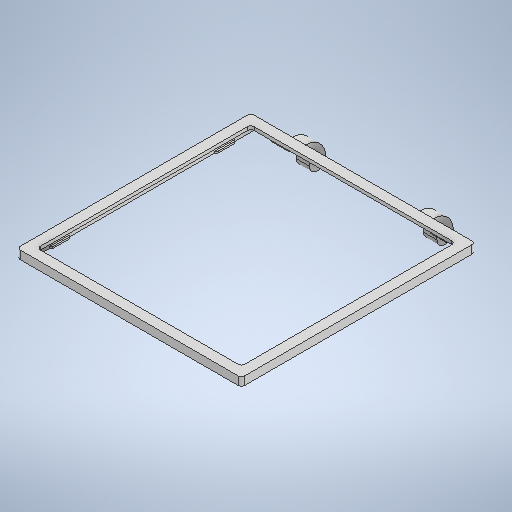
# Autodesk Inventor part: Pieza4
Saved by Autodesk Inventor 2025.1 (Build 291241000, 241)
## iProperties
Created: 2024-08-13
Part Number: Pieza4
Material: Genérico
Document SubType Name: Modeling
Designer: andre
Density: 1 g/cm^3
Appearance: Valor por defecto
Author: andre
Autodesk Inventor part; units mm, degrees
ref_plane "YZ Plane" through (0, 0, 0) normal (1, 0, 0) x (0, 1, 0)
ref_plane "XZ Plane" through (0, 0, 0) normal (0, 1, 0) x (-1, 0, 0)
ref_plane "XY Plane" through (0, 0, 0) normal (0, 0, 1) x (1, 0, 0)
sketch "Boceto1" plane through (0, 0, 0) normal (0, 1, 0) x (-1, 0, 0)
  line L0 (2, 0) -> (132.4, 0)
  line L1 (134.4, -2) -> (134.4, -138)
  line L2 (132.4, -140) -> (2, -140)
  line L3 (0, -138) -> (0, -2)
  arc A0 (134.4, -2) -> (132.4, 0) centre (132.4, -2) ccw
  arc A1 (132.4, -140) -> (134.4, -138) centre (132.4, -138) ccw
  arc A2 (0, -138) -> (2, -140) centre (2, -138) ccw
  arc A3 (2, 0) -> (0, -2) centre (2, -2) ccw
  line L4 (126.4, -6) -> (8, -6)
  line L5 (6, -8) -> (6, -132)
  line L6 (8, -134) -> (126.4, -134)
  line L7 (128.4, -132) -> (128.4, -8)
  arc A4 (8, -6) -> (6, -8) centre (8, -8) ccw
  arc A5 (6, -132) -> (8, -134) centre (8, -132) ccw
  arc A6 (126.4, -134) -> (128.4, -132) centre (126.4, -132) ccw
  arc A7 (128.4, -8) -> (126.4, -6) centre (126.4, -8) ccw
  line L8 (67.2, -140) -> (67.2, 0) construction
  line L9 (134.4, -140) -> (109.4, -140) construction
  line L10 (109.4, -140) -> (101.4, -140) construction
  line L11 (101.4, -140) -> (101.4, -152)
  line L12 (101.4, -152) -> (109.4, -152)
  line L13 (109.4, -152) -> (109.4, -140)
  line L14 (0, -140) -> (25, -140) construction
  line L15 (25, -140) -> (33, -140) construction
  line L16 (33, -140) -> (33, -152)
  line L17 (33, -152) -> (25, -152)
  line L18 (25, -152) -> (25, -140)
  point P0 (0, 0)
  point P1 (134.4, 0)
  point P2 (25, -140)
  point P3 (101.4, -140)
  dimension "d0" = 134.4
  dimension "d1" = 140
  dimension "d2" = 2
  dimension "d3" = 6
  dimension "d4" = 2
  dimension "d7" = 25
  dimension "d8" = 8
  dimension "d9" = 12
  constraints: 38 end point, 16 point on circle, 16 tangent, 9 point on line, 8 centre point, 6 equal radius, 6 parallel, 4 symmetric about line, 3 perpendicular, 2 horizontal, 2 midpoint, 3 other
  measures "d0" distance of L9.start L14.start
  measures "d1" distance of point (134.4, 0) L9.start
  measures "d2" radius of A0
  measures "d3" distance between parallel lines of L0 L4
  measures "d4" radius of A4
  measures "d7" distance of L9.start L9.end
  measures "d8" distance of L12.end L11.end
  measures "d9" distance of L11.end L10.end
extrude "Extrusión1" add sketch "Boceto1" along normal blind 5
sketch "Boceto2" plane through (0, 0, 0) normal (0, -1, 0) x (1, 0, 0)
  line L0 (-25, -140) -> (-25, -152) projected
  line L1 (-33, -140) -> (-101.4, -140) projected
  line L2 (-25, -152) -> (-33, -152)
  line L3 (-33, -152) -> (-33, -140)
  line L4 (-33, -140) -> (-25, -140)
  line L5 (-25, -140) -> (-25, -152)
  line L6 (-101.4, -152) -> (-109.4, -152) projected
  line L7 (-109.4, -152) -> (-101.4, -152)
  line L8 (-101.4, -152) -> (-101.4, -140)
  line L9 (-101.4, -140) -> (-109.4, -140)
  line L10 (-109.4, -140) -> (-109.4, -152)
  line L11 (-109.4, -140) -> (-101.4, -140)
  line L12 (-101.4, -140) -> (-101.4, -136)
  line L13 (-101.4, -136) -> (-109.4, -136)
  line L14 (-109.4, -136) -> (-109.4, -140)
  line L15 (-33, -140) -> (-25, -140)
  line L16 (-25, -140) -> (-25, -136)
  line L17 (-25, -136) -> (-33, -136)
  line L18 (-33, -136) -> (-33, -140)
  point P0 (0, 0)
  dimension "d18" = 4
  dimension "d19" = 8
  dimension "d20" = 4
  constraints: 32 end point, 8 parallel, 4 horizontal, 4 perpendicular
  measures "d18" distance of L12.end L11.end
  measures "d19" distance of L17.end L16.end
  measures "d20" distance of L16.end L15.end
extrude "Extrusión2" add sketch "Boceto2" along normal blind 18
sketch "Boceto3" plane through (-109.4, 5, -152) normal (-1, 0, 0) x (0, 0, 1)
  line L0 (14, -5) -> (12, -5) construction
  line L1 (0, -23) -> (0, 0) projected
  line L2 (12, -5) -> (0, -5) construction
  line L3 (0, -5) -> (0, -12) construction
  line L4 (12, -12) -> (12, -5) construction
  circle A0 centre (5, -12) radius 2.125
  circle A1 centre (5, -12) radius 4.875 construction
  arc A2 (0.125, -12) -> (9.875, -12) centre (5, -12) ccw
  line L5 (0.125, -12) -> (0.125, 0) construction
  line L6 (12, 0) -> (0, 0) construction
  line L7 (12, -5) -> (12, 0) construction
  line L8 (9.8743, -12.0803) -> (9.8743, -5) construction
  line L9 (12, -5) -> (5, -5) construction
  line L10 (5, -5) -> (5, -12) construction
  line L11 (5, -12) -> (12, -12) construction
  line L12 (12, -12) -> (12, -5) construction
  line L13 (14, -5) -> (14, -23) construction
  line L14 (16, -23) -> (0, -23) projected
  line L15 (12, -5) -> (14, -5) construction
  line L16 (14, -5) -> (14, -7) construction
  line L17 (14, -7) -> (12, -7) construction
  line L18 (12, -7) -> (12, -5) construction
  arc A3 (14, -5) -> (12, -7) centre (14, -7) ccw construction
  line L19 (14, 0) -> (150, 0) projected
  line L20 (12, 0) -> (14, 0)
  arc A4 (12, 0) -> (0.125, -12) centre (12, -11.8757) ccw
  line L21 (14, -5) -> (16, -5)
  arc A5 (14, -5) -> (9.8743, -9.1856) centre (14, -9.1261) ccw
  line L22 (9.8743, -12.0803) -> (9.8743, -9.1856)
  line L23 (0.125, 0) -> (14, 0)
  line L24 (14, 0) -> (14, -23)
  line L25 (14, -23) -> (0, -23)
  line L26 (16, -23) -> (14, -23)
  line L27 (14, -23) -> (14, -5)
  line L28 (14, -5) -> (16, -5)
  line L29 (16, -5) -> (16, -23)
  line L30 (0.125, 0) -> (-6.5711, 0)
  line L31 (-6.5711, 0) -> (-6.5711, -23)
  line L32 (-6.5711, -23) -> (16, -23)
  point P0 (152, -5)
  point P1 (9.8743, -9.1856)
  point P2 (9.8743, -12.0803)
  point P3 (0, -10.3846)
  point P4 (0, -13.125)
  point P5 (12, 0)
  point P6 (0, 0)
  point P7 (14, -5)
  point P8 (14, -5)
  dimension "d13" = 4.25
  dimension "d14" = 2.75
  dimension "d16" = 7
  dimension "d17" = 7
  dimension "d21" = 2
  constraints: 54 end point, 11 point on circle, 8 parallel, 7 perpendicular, 6 centre point, 6 horizontal, 6 point on line, 3 coincident, 3 vertical, 2 collinear, 2 tangent, 1 concentric
  measures "d13" diameter of A0
  measures "d14" radial gap between concentric circles of A0 A1
  measures "d16" distance of L11.end L10.end
  measures "d17" distance of L10.end L9.end
  measures "d21" distance of L16.end L17.end
extrude "Extrusión3" cut sketch "Boceto3" against normal blind 150 contours L1 L30 L23 A4 A2 L22 A5 L24 L14 | L24 L21 L29 L14 | A0
sketch "Boceto4" plane through (0, 0, 0) normal (0, -1, 0) x (1, 0, 0)
  line L0 (0, 0) -> (-132, 0)
  line L1 (-132, 0) -> (-132, -140)
  line L2 (-132, -140) -> (0, -140)
  line L3 (0, -140) -> (0, 0)
  line L4 (-2.5, -2.5) -> (-129.5, -2.5)
  line L5 (-129.5, -2.5) -> (-129.5, -137.5)
  line L6 (-129.5, -137.5) -> (-2.5, -137.5)
  line L7 (-2.5, -137.5) -> (-2.5, -2.5)
  dimension "d27" = 132
  dimension "d28" = 140
  dimension "d29" = 2.5
  constraints: 16 end point, 4 parallel, 2 perpendicular, 1 horizontal, 3 other
  measures "d27" distance of L2.end L1.end
  measures "d28" distance of L1.end L0.end
  measures "d29" distance between parallel lines of L3 L7
extrude "Extrusión4" cut sketch "Boceto4" against normal blind 3 contours L7 L6 L5 L4
sketch "Boceto5" plane through (0, 0, 0) normal (0, -1, 0) x (1, 0, 0)
  line L0 (-129.5, -137.5) -> (-129.5, -2.5) projected
  line L1 (-2.5, -2.5) -> (-2.5, -137.5) projected
  line L2 (-129.5, -137.5) -> (-2.5, -137.5)
  line L3 (-2.5, -137.5) -> (-2.5, -2.5)
  line L4 (-2.5, -2.5) -> (-129.5, -2.5)
  line L5 (-129.5, -2.5) -> (-129.5, -137.5)
  line L6 (-2.5, -137.5) -> (-129.5, -137.5) projected
  line L7 (-66, -137.5) -> (-66, -2.5) construction
  line L8 (-33, -140) -> (-101.4, -140) construction
  line L9 (-2.5, -70) -> (-129.5, -70) construction
  line L10 (-118.5, -137.5) -> (-107.5, -137.5) construction
  line L11 (-118.5, -137.5) -> (-108.5, -137.5) construction
  line L12 (-108.5, -137.5) -> (-108.5, -136.5) construction
  line L13 (-108.5, -136.5) -> (-118.5, -136.5) construction
  line L14 (-118.5, -136.5) -> (-118.5, -137.5) construction
  line L15 (-118.5, -137.5) -> (-119.5, -137.5) construction
  line L16 (-119.5, -137.5) -> (-118.5, -136.5) construction
  line L17 (-108.5, -137.5) -> (-107.5, -137.5) construction
  line L18 (-107.5, -137.5) -> (-108.5, -136.5) construction
  line L19 (-107.5, -137.5) -> (-108.5, -136.5)
  line L20 (-118.5, -136.5) -> (-119.5, -137.5)
  line L21 (-118.5, -136.5) -> (-108.5, -136.5)
  line L22 (-129.5, -124.5) -> (-128.5, -124.5) construction
  line L23 (-128.5, -124.5) -> (-128.5, -114.5) construction
  line L24 (-128.5, -114.5) -> (-129.5, -114.5) construction
  line L25 (-129.5, -114.5) -> (-129.5, -124.5) construction
  line L26 (-129.5, -124.5) -> (-129.5, -125.5) construction
  line L27 (-129.5, -125.5) -> (-128.5, -124.5) construction
  line L28 (-129.5, -114.5) -> (-129.5, -113.5) construction
  line L29 (-129.5, -113.5) -> (-128.5, -114.5) construction
  line L30 (-129.5, -125.5) -> (-128.5, -124.5)
  line L31 (-128.5, -114.5) -> (-128.5, -124.5)
  line L32 (-129.5, -113.5) -> (-128.5, -114.5)
  line L33 (-107.5, -137.5) -> (-119.5, -137.5)
  line L34 (-129.5, -125.5) -> (-129.5, -113.5)
  line L35 (-118.5, -2.5) -> (-107.5, -2.5) construction
  line L36 (-118.5, -2.5) -> (-108.5, -2.5) construction
  line L37 (-108.5, -2.5) -> (-108.5, -3.5) construction
  line L38 (-108.5, -3.5) -> (-118.5, -3.5) construction
  line L39 (-118.5, -3.5) -> (-118.5, -2.5) construction
  line L40 (-118.5, -2.5) -> (-119.5, -2.5) construction
  line L41 (-119.5, -2.5) -> (-118.5, -3.5) construction
  line L42 (-108.5, -2.5) -> (-107.5, -2.5) construction
  line L43 (-107.5, -2.5) -> (-108.5, -3.5) construction
  line L44 (-107.5, -2.5) -> (-108.5, -3.5)
  line L45 (-118.5, -3.5) -> (-119.5, -2.5)
  line L46 (-118.5, -3.5) -> (-108.5, -3.5)
  line L47 (-129.5, -15.5) -> (-128.5, -15.5) construction
  line L48 (-128.5, -15.5) -> (-128.5, -25.5) construction
  line L49 (-128.5, -25.5) -> (-129.5, -25.5) construction
  line L50 (-129.5, -25.5) -> (-129.5, -15.5) construction
  line L51 (-129.5, -15.5) -> (-129.5, -14.5) construction
  line L52 (-129.5, -14.5) -> (-128.5, -15.5) construction
  line L53 (-129.5, -25.5) -> (-129.5, -26.5) construction
  line L54 (-129.5, -26.5) -> (-128.5, -25.5) construction
  line L55 (-129.5, -14.5) -> (-128.5, -15.5)
  line L56 (-128.5, -25.5) -> (-128.5, -15.5)
  line L57 (-129.5, -26.5) -> (-128.5, -25.5)
  line L58 (-107.5, -2.5) -> (-119.5, -2.5)
  line L59 (-129.5, -14.5) -> (-129.5, -26.5)
  line L60 (-2.5, -137.5) -> (-2.5, -2.5)
  line L61 (-2.5, -2.5) -> (-2.5, -137.5)
  line L62 (-13.5, -137.5) -> (-24.5, -137.5) construction
  line L63 (-13.5, -137.5) -> (-23.5, -137.5) construction
  line L64 (-23.5, -137.5) -> (-23.5, -136.5) construction
  line L65 (-23.5, -136.5) -> (-13.5, -136.5) construction
  line L66 (-13.5, -136.5) -> (-13.5, -137.5) construction
  line L67 (-13.5, -137.5) -> (-12.5, -137.5) construction
  line L68 (-12.5, -137.5) -> (-13.5, -136.5) construction
  line L69 (-23.5, -137.5) -> (-24.5, -137.5) construction
  line L70 (-24.5, -137.5) -> (-23.5, -136.5) construction
  line L71 (-24.5, -137.5) -> (-23.5, -136.5)
  line L72 (-13.5, -136.5) -> (-12.5, -137.5)
  line L73 (-13.5, -136.5) -> (-23.5, -136.5)
  line L74 (-2.5, -124.5) -> (-3.5, -124.5) construction
  line L75 (-3.5, -124.5) -> (-3.5, -114.5) construction
  line L76 (-3.5, -114.5) -> (-2.5, -114.5) construction
  line L77 (-2.5, -114.5) -> (-2.5, -124.5) construction
  line L78 (-2.5, -124.5) -> (-2.5, -125.5) construction
  line L79 (-2.5, -125.5) -> (-3.5, -124.5) construction
  line L80 (-2.5, -114.5) -> (-2.5, -113.5) construction
  line L81 (-2.5, -113.5) -> (-3.5, -114.5) construction
  line L82 (-2.5, -125.5) -> (-3.5, -124.5)
  line L83 (-3.5, -114.5) -> (-3.5, -124.5)
  line L84 (-2.5, -113.5) -> (-3.5, -114.5)
  line L85 (-24.5, -137.5) -> (-12.5, -137.5)
  line L86 (-2.5, -125.5) -> (-2.5, -113.5)
  line L87 (-3.5, -25.5) -> (-2.5, -25.5) construction
  line L88 (-2.5, -26.5) -> (-3.5, -25.5) construction
  line L89 (-2.5, -26.5) -> (-3.5, -25.5)
  line L90 (-2.5, -15.5) -> (-3.5, -15.5) construction
  line L91 (-2.5, -25.5) -> (-2.5, -15.5) construction
  line L92 (-2.5, -14.5) -> (-3.5, -15.5) construction
  line L93 (-2.5, -14.5) -> (-3.5, -15.5)
  line L94 (-2.5, -14.5) -> (-2.5, -26.5)
  line L95 (-2.5, -25.5) -> (-2.5, -26.5) construction
  line L96 (-3.5, -15.5) -> (-3.5, -25.5) construction
  line L97 (-3.5, -25.5) -> (-3.5, -15.5)
  line L98 (-2.5, -15.5) -> (-2.5, -14.5) construction
  line L99 (-13.5, -2.5) -> (-24.5, -2.5) construction
  line L100 (-13.5, -2.5) -> (-12.5, -2.5) construction
  line L101 (-12.5, -2.5) -> (-13.5, -3.5) construction
  line L102 (-13.5, -3.5) -> (-12.5, -2.5)
  line L103 (-23.5, -3.5) -> (-13.5, -3.5) construction
  line L104 (-13.5, -3.5) -> (-23.5, -3.5)
  line L105 (-13.5, -2.5) -> (-23.5, -2.5) construction
  line L106 (-23.5, -2.5) -> (-23.5, -3.5) construction
  line L107 (-24.5, -2.5) -> (-12.5, -2.5)
  line L108 (-23.5, -2.5) -> (-24.5, -2.5) construction
  line L109 (-24.5, -2.5) -> (-23.5, -3.5) construction
  line L110 (-24.5, -2.5) -> (-23.5, -3.5)
  line L111 (-13.5, -3.5) -> (-13.5, -2.5) construction
  point P0 (0, 0)
  point P1 (-101.4, 0)
  point P2 (-30.6, 0)
  dimension "d32" = 11
  dimension "d33" = 13
  dimension "d36" = 10
  dimension "d37" = 1
  dimension "d38" = 1
  dimension "d40" = 1
  dimension "d41" = 1
  dimension "d42" = 10
  dimension "d43" = 1
  dimension "d44" = 1
  constraints: 216 end point, 40 symmetric about line, 8 point on line, 7 collinear, 6 parallel, 6 perpendicular, 4 horizontal, 4 midpoint, 1 vertical
  measures "d32" distance of L10.start L0.start
  measures "d33" distance of L22.start L0.start
  measures "d36" distance of L13.end L12.end
  measures "d37" distance of L12.end L11.end
  measures "d38" distance of L10.start L15.end
  measures "d40" distance of L11.end L10.end
  measures "d41" distance of L24.end L23.end
  measures "d42" distance of L23.end L22.end
  measures "d43" distance of L22.start L26.end
  measures "d44" distance of L24.end L28.end
extrude "Extrusión5" add sketch "Boceto5" against normal blind 1 contours L0 L32 L31 L30 | L20 L21 L19 L2 | L0 L55 L56 L57 | L71 L73 L72 L2 | L4 L44 L46 L45 | L82 L83 L84 L1 | L4 L102 L104 L110 | L89 L97 L93 L1
